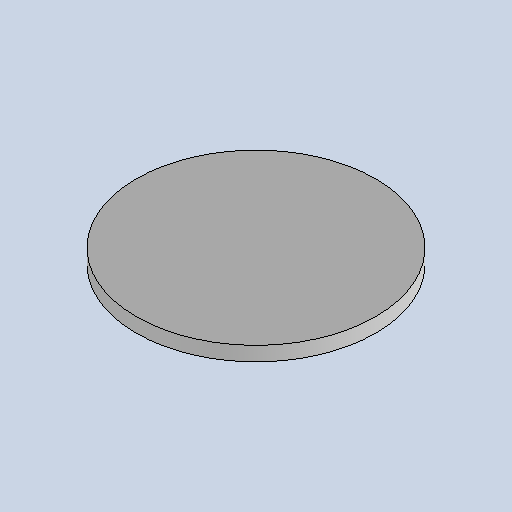
# Autodesk Inventor part: GNH 082 leg plate
Saved by Autodesk Inventor 2025.1 (Build 291241020, 241B)
## iProperties
Created: 2025-03-06
Part Number: GNH 082 leg plate
Material: Stainless Steel
Document SubType Name: Sheet Metal
Designer: user
Density: 8 g/cm^3
Flat Pattern Width: 5 cm
Flat Pattern Length: 5 cm
Flat Pattern Area: 25 cm^2
Sheet Metal Rule: AISI304 3mm Die 32
Sheet Metal Width: 50.000 mm
Sheet Metal Length: 50.000 mm
Sheet Metal Area: 2500.000 mm^2
Appearance: Default
Author: user
Autodesk Inventor part; units mm, degrees
ref_plane "YZ Plane" through (0, 0, 0) normal (1, 0, 0) x (0, 1, 0)
ref_plane "XZ Plane" through (0, 0, 0) normal (0, 1, 0) x (-1, 0, 0)
ref_plane "XY Plane" through (0, 0, 0) normal (0, 0, 1) x (1, 0, 0)
sketch "Sketch1" plane through (0, 0, 0) normal (0, 0, 1) x (1, 0, 0)
  circle A0 centre (0, 0) radius 25
  dimension "d7" = 50
  measures "d7" diameter of A0
extrude "Plate1" add sketch "Sketch1" along normal blind 3
feature "Corner Round2" [suppressed]
equation "\"d2\" = Thickness"
equation "\"BendReliefWidth\" = Thickness"
equation "\"BendReliefDepth\" = 0.5 * Thickness"
equation "\"CornerReliefSize\" = 4 * Thickness"
equation "\"MinimumRemnant\" = 2 * Thickness"
equation "\"TransitionRadius\" = BendRadius"
equation "\"JacobiRadiusSize\" = BendRadius"
equation "\"GapSize\" = Thickness"
equation "\"Thickness\" = 3"
equation "\"BendRadius\" = 5"
body "Solid1"
